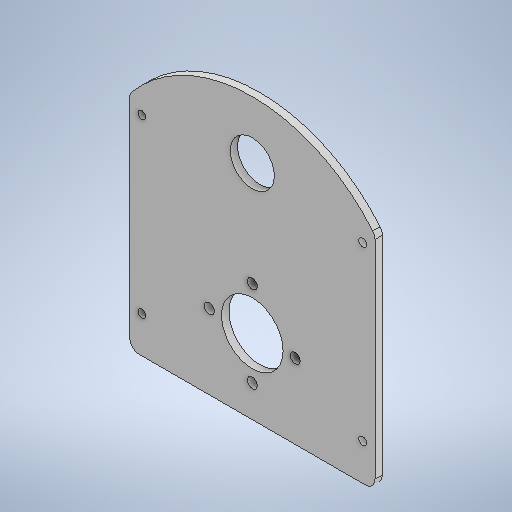
# Autodesk Inventor part: aaa_plate_motor
Saved by Autodesk Inventor 2025.1 (Build 291241000, 241)
## iProperties
Created: 2024-12-20
Part Number: aaa_plate_motor
Material: 一般
Document SubType Name: Modeling
Designer: yuki0520
Density: 1 g/cm^3
Appearance: 既定
Author: yuki0520
Autodesk Inventor part; units mm, degrees
ref_plane "YZ Plane" through (0, 0, 0) normal (1, 0, 0) x (0, 1, 0)
ref_plane "XZ Plane" through (0, 0, 0) normal (0, 1, 0) x (-1, 0, 0)
ref_plane "XY Plane" through (0, 0, 0) normal (0, 0, 1) x (1, 0, 0)
sketch "スケッチ1" plane through (0, 0, 0) normal (0, 0, 1) x (1, 0, 0)
  point P0 (0, 0)
sketch "スケッチ2" plane through (0, 0, 0) normal (0, 0, 1) x (1, 0, 0)
  line L0 (50, -40) -> (-50, -40)
  line L1 (-50, -40) -> (-50, 40)
  line L2 (-50, 40) -> (50, 40)
  line L3 (50, 40) -> (50, -40)
  line L4 (50, -40) -> (-50, 40) construction
  line L5 (-50, -40) -> (50, 40) construction
  circle A0 centre (0, -19.5) radius 12.55
  circle A1 centre (0, -19.5) radius 17.5
  circle A2 centre (17.5, -19.5) radius 2.05
  circle A3 centre (0, -2) radius 2.05
  circle A4 centre (-17.5, -19.5) radius 2.05
  circle A5 centre (0, -37) radius 2.05
  line L6 (45, 35) -> (-45, 35)
  line L7 (-45, 35) -> (-45, -35)
  line L8 (-45, -35) -> (45, -35)
  line L9 (45, -35) -> (45, 35)
  line L10 (-45, 35) -> (-45, 35) construction
  line L11 (-46.6, 35) -> (-46.6, 35)
  line L12 (-43.4, 35) -> (-43.4, 35)
  arc A6 (-43.4, 35) -> (-46.6, 35) centre (-45, 35) ccw
  arc A7 (-46.6, 35) -> (-43.4, 35) centre (-45, 35) ccw
  line L13 (-45, 35) -> (-45, 35) construction
  line L14 (-45, -35) -> (-45, -35) construction
  line L15 (-43.4, -35) -> (-43.4, -35)
  line L16 (-46.6, -35) -> (-46.6, -35)
  arc A8 (-46.6, -35) -> (-43.4, -35) centre (-45, -35) ccw
  arc A9 (-43.4, -35) -> (-46.6, -35) centre (-45, -35) ccw
  line L17 (-45, -35) -> (-45, -35) construction
  line L18 (45, 35) -> (45, 35) construction
  line L19 (43.4, 35) -> (43.4, 35)
  line L20 (46.6, 35) -> (46.6, 35)
  arc A10 (46.6, 35) -> (43.4, 35) centre (45, 35) ccw
  arc A11 (43.4, 35) -> (46.6, 35) centre (45, 35) ccw
  line L21 (45, 35) -> (45, 35) construction
  line L22 (45, -35) -> (45, -35) construction
  line L23 (46.6, -35) -> (46.6, -35)
  line L24 (43.4, -35) -> (43.4, -35)
  arc A12 (43.4, -35) -> (46.6, -35) centre (45, -35) ccw
  arc A13 (46.6, -35) -> (43.4, -35) centre (45, -35) ccw
  line L25 (45, -35) -> (45, -35) construction
  line L26 (-50, -19.5) -> (50, -19.5)
  circle A14 centre (0, -19.5) radius 9
  circle A15 centre (0, -19.5) radius 39
  line L27 (-50, 0) -> (50, 0)
  line L28 (50, 0) -> (50, -50)
  line L29 (50, -50) -> (-50, -50)
  line L30 (-50, -50) -> (-50, 0)
  arc A16 (50, 40) -> (-50, 40) centre (0, 0) ccw
  circle A17 centre (0, 40.5) radius 15
  line L31 (0, 64.0312) -> (0, -19.5)
  circle A18 centre (0, 40.5) radius 9
  circle A19 centre (0, 55.5) radius 1.55
  circle A20 centre (0, 25.5) radius 1.55
  point P0 (-98, -19.5)
  point P1 (-45, 35)
  point P2 (-45, -35)
  point P3 (45, 35)
  point P4 (45, -35)
  point P5 (0, 40)
  point P6 (0.45, -35)
  point P7 (-0.45, -35)
  point P8 (-50, -40)
  point P9 (43.4, 35)
  point P10 (-46.6, 35)
  point P11 (-43.4, 35)
  point P12 (-43.4, -35)
  point P13 (-46.6, -35)
  point P14 (-0.45, 0)
  point P15 (0.45, 0)
  dimension "d9" = 35
  dimension "d0" = 100
  dimension "d1" = 80
  dimension "d6" = 25.1
  dimension "d10" = 4.1
  dimension "d13" = 360
  dimension "d21" = 5
  dimension "d22" = 0
  dimension "d23" = 90
  dimension "d24" = 3.2
  dimension "d25" = 0
  dimension "d26" = 90
  dimension "d27" = 3.2
  dimension "d28" = 0
  dimension "d29" = 90
  dimension "d30" = 3.2
  dimension "d31" = 0
  dimension "d32" = 90
  dimension "d33" = 3.2
  dimension "d36" = 20.5
  dimension "d37" = 18
  dimension "d38" = 78
  dimension "d46" = 50
  dimension "d47" = 30
  dimension "d48" = 60
  dimension "d49" = 18
  dimension "d50" = 3.1
  dimension "d51" = 3.1
  constraints: 72 end point, 21 point on circle, 20 centre point, 16 tangent, 10 midpoint, 10 parallel, 8 perpendicular, 7 point on line, 6 horizontal, 5 collinear, 4 coincident, 1 concentric, 1 horizontal alignment, 1 vertical, 14 other
  measures "d0" distance of L1.end L2.end
  measures "d1" distance of L0.end L1.end
  measures "d6" diameter of A0
  measures "d10" diameter of A2
  measures "d21" distance between parallel lines of L2 L6
  measures "d22" distance of L6.end L10.end
  measures "d23" angle of L10 L13
  measures "d24" diameter of A7
  measures "d25" distance of L7.end L14.end
  measures "d26" angle of L17 L14
  measures "d27" diameter of A9
  measures "d28" distance of L6.start L18.end
  measures "d29" angle of L18 L21
  measures "d30" diameter of A11
  measures "d31" distance of L8.end L22.end
  measures "d32" angle of L25 L22
  measures "d33" diameter of A13
  measures "d36" distance between parallel lines of L0 L26
  measures "d37" diameter of A14
  measures "d38" diameter of A15
  measures "d46" distance of L27.end L28.end
  measures "d47" diameter of A17
  measures "d48" distance of A14.centre A17.centre
  measures "d49" diameter of A18
  measures "d50" diameter of A19
  measures "d51" diameter of A20
extrude "押し出し1" add sketch "スケッチ2" along normal blind 3 contours L28 L29 A15 L0 | L0 A15 L8 A12 A13 L9 L26 L3 | A15 L29 L0 | L0 A15 L8 A1 A5 | L26 L9 L27 L3 | A15 L29 L30 L0 | L0 L1 L26 L7 A9 A8 L8 A15 | A15 L26 L9 A13 L8 | L8 A1 A2 L26 A15 | L27 L9 A11 A10 L6 A17 L2 L3 | L26 A15 L27 L9 | A15 L26 A4 A1 L8 | L8 A9 L7 L26 A15 | L8 A5 A1 A4 L26 A0 A2 | A1 A5 L8 | L26 A2 A1 A3 L27 A15 | L2 A17 A19 L31 A16 | L27 A15 L31 A20 A17 L6 A11 L9 | L1 L27 L7 L26 | L8 A5 A1 | A15 L27 A3 A1 A4 L26 | L26 L7 L27 A15 | L8 A5 | L27 A3 L31 A15 | A17 L6 A18 L2 | L2 A18 L31 A19 A17 | L31 A19 A17 L2 A16 | L1 L2 A17 L6 A6 A7 L7 L27 | L27 L7 A7 L6 A17 A20 L31 A15 | A15 L31 A3 L27 | L26 A0 L31 A3 A1 A2 | L27 L31 A3 | A17 A20 L31 A18 L6 | A19 A17 L31 | L31 A17 A19 | A4 A1 A3 L31 A0 L26 | A3 L31 L27 | A20 A17 L31 | L31 A17 A20 | A17 L31 A20 | A19 L31 A17 | A17 A19 L31 A18 L2 | L2 A18 L6 A17 | L31 A19 A17 | A17 A20 L31 | A17 L6 A18 L31 A20 picked at (5.1824, -35.4142) picked at (-5.1824, -35.4142)
fillet "フィレット1" radius 4 4 edges at (50, 40, 1.5) (-50, 40, 1.5) (50, -50, 1.5) (-50, -50, 1.5)
equation "\"d27\" = d24"
equation "\"d30\" = d24"
equation "\"d33\" = d24"
